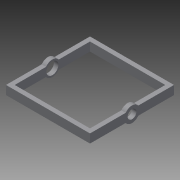
# Autodesk Inventor part: joystick_outer
Saved by Autodesk Inventor 2015 (Build 190159000, 159)
## iProperties
Created: 2015-12-08
Part Number: joystick_outer
Material: Generic
Document SubType Name: Modeling
Designer: boztalay
Density: 1 g/cm^3
Appearance: Default
Author: boztalay
Autodesk Inventor part; units mm, degrees
ref_plane "YZ Plane" through (0, 0, 0) normal (1, 0, 0) x (0, 1, 0)
ref_plane "XZ Plane" through (0, 0, 0) normal (0, 1, 0) x (-1, 0, 0)
ref_plane "XY Plane" through (0, 0, 0) normal (0, 0, 1) x (1, 0, 0)
sketch "Sketch1" plane through (0, 0, 0) normal (0, 1, 0) x (-1, 0, 0)
  line L0 (-54.61, 54.61) -> (54.61, 54.61)
  line L1 (54.61, 54.61) -> (54.61, -54.61)
  line L2 (54.61, -54.61) -> (-54.61, -54.61)
  line L3 (-54.61, -54.61) -> (-54.61, 54.61)
  line L4 (-54.61, 54.61) -> (54.61, -54.61) construction
  line L5 (54.61, 54.61) -> (-54.61, -54.61) construction
  line L6 (-60.96, 60.96) -> (60.96, 60.96)
  line L7 (60.96, 60.96) -> (60.96, -60.96)
  line L8 (60.96, -60.96) -> (-60.96, -60.96)
  line L9 (-60.96, -60.96) -> (-60.96, 60.96)
  line L10 (-60.96, 60.96) -> (60.96, -60.96) construction
  line L11 (60.96, 60.96) -> (-60.96, -60.96) construction
  point P0 (0, 0)
  dimension "d0" = 109.22
  dimension "d1" = 109.22
  dimension "d2" = 121.92
  dimension "d3" = 121.92
  constraints: 24 end point, 4 midpoint, 4 parallel, 2 horizontal, 2 perpendicular
  measures "d0" distance of L0.end L1.end
  measures "d1" distance of L1.end L2.end
  measures "d2" distance of L6.end L7.end
  measures "d3" distance of L7.end L8.end
extrude "Extrusion1" add sketch "Sketch1" along normal blind 12.7
sketch "Sketch2" plane through (-60.96, 0, -60.96) normal (-1, 0, 0) x (0, 0, 1)
  circle A0 centre (60.96, 6.35) radius 11.1125
  point P0 (60.96, 0)
  dimension "d6" = 22.225
  constraints: 1 centre point
  measures "d6" diameter of A0
extrude "Extrusion2" add sketch "Sketch2" against normal up to surface (6.35 mm away)
sketch "Sketch3" plane through (-60.96, 0, -60.96) normal (-1, 0, 0) x (0, 0, 1)
  circle A0 centre (60.96, 6.35) radius 8.7313
  point P0 (60.96, 0)
  dimension "d9" = 17.4625
  constraints: 1 centre point
  measures "d9" diameter of A0
extrude "Extrusion3" cut sketch "Sketch3" against normal up to next
sketch "Sketch4" plane through (60.96, 0, 60.96) normal (1, 0, 0) x (0, 0, -1)
  circle A0 centre (60.96, 6.35) radius 11.1125
  point P0 (60.96, 0)
  constraints: 1 centre point
extrude "Extrusion4" add sketch "Sketch4" against normal up to surface (6.35 mm away)
sketch "Sketch5" plane through (60.96, 0, 60.96) normal (1, 0, 0) x (0, 0, -1)
  circle A0 centre (60.96, 6.35) radius 6.35
  point P0 (60.96, 0)
  dimension "d14" = 12.7
  constraints: 1 centre point
  measures "d14" diameter of A0
extrude "Extrusion5" cut sketch "Sketch5" against normal up to next
body "Solid1"
